Autodesk Inventor part; units mm, degrees
(part 3 of 3)
emboss "Emboss1" sketch "Sketch3" operation cut depth 0.1 direction (0, 1, 0) contours L352 L341 L342 L343 L344 L345 L346 L347 L348 L349 L350 L351 | S1 L0 L1 L2 S2 S3 S0 | L17 L6 L7 L8 L9 L10 L11 L12 L13 L14 L15 L16 | L22 L23 L24 L25 L26 L27 L28 L29 L30 L31 L32 L33 | L51 L52 L53 L54 L55 L56 L57 L58 L59 L60 L61 L62 | L63 L64 L65 L66 L67 L68 L69 L70 L71 L72 L73 L74 | L109 L98 L99 L100 L101 L102 L103 L104 L105 L106 L107 L108 | L128 L117 L118 L119 L120 L121 L122 L123 L124 L125 L126 L127 | L155 L144 L145 L146 L147 L148 L149 L150 L151 L152 L153 L154 | L167 L156 L157 L158 L159 L160 L161 L162 L163 L164 L165 L166 | L185 L186 L187 L188 L189 L190 L191 L192 L193 L194 L195 L196 | L218 L207 L208 L209 L210 L211 L212 L213 L214 L215 L216 L217 | L230 L219 L220 L221 L222 L223 L224 L225 L226 L227 L228 L229 | L242 L243 L244 L245 L246 L247 L248 L249 L250 L251 L252 L253 | L308 L297 L298 L299 L300 L301 L302 L303 L304 L305 L306 L307 | A0 L333 L334 L335 L336 L337 L338 L339 | A0 L313 L314 L315 L316 L317 L318 L319 | S155 S156 S157 S158 S159 L377 L378 S160 S161 S162 S163 S164 S153 S154 A0 | A0 S154 S155 | S152 S137 A0 | A0 S137 S138 S139 S140 S141 S142 L309 L310 S143 S144 S145 S146 S147 S148 S149 S150 L311 L312 S151 S152 | S132 S133 A0 | A0 S133 L290 L291 S134 S135 S136 L292 L293 L294 L295 L296 S132 | S8 L18 L19 S9 S10 S11 S12 S13 S14 S15 S16 L20 L21 S17 S18 S19 S20 S21 S22 S23 A0 | A0 S23 S8 | S120 S121 A0 | A0 S121 S122 S123 S124 S125 S118 S119 S120 | S24 S25 S26 S27 S28 S29 L34 L35 S30 S31 S32 S33 S34 S35 L36 L37 L38 L39 L40 S36 S37 A0 | A0 S37 S24 | S102 S89 A0 | A0 S89 S90 S91 S92 S93 S94 L264 L265 S95 S96 S97 S98 S99 S100 L266 L267 L268 L269 L270 S101 S102 | L112 L113 L114 L115 L116 L110 A0 | S81 S68 A0 | A0 S68 S69 S70 S71 S72 S73 L178 L179 S74 S75 S76 S77 S78 S79 L180 L181 L182 L183 L184 S80 S81 | S52 L140 L141 S53 S54 S55 S56 S57 S58 S59 S60 L142 L143 S61 S62 S63 S64 S65 S66 S67 A0 | A0 S67 S52 | L41 L42 L43 L44 L45 L46 L47 L48 L49 L50 | L75 L76 L77 L78 | L79 L80 L81 L82 | L83 L84 L85 L86 | L87 L88 L89 L90 L91 L92 L93 S38 S39 S40 L94 | L129 L130 L131 L132 L133 L134 L135 S45 S46 S47 L136 | L168 L169 L170 L171 L172 L173 L174 L175 L176 L177 | L197 L198 L199 L200 L201 L202 L203 L204 L205 L206 | L231 L232 L233 L234 L235 L236 L237 S82 S83 S84 L238 | L254 L255 L256 L257 L258 L259 L260 L261 L262 L263 | S103 S104 L271 L272 L273 L274 L275 S105 S106 | L279 L280 L281 L282 L283 L284 L285 S111 S112 S113 L286 | L321 L322 L323 L324 | L325 L326 L327 L328 | L329 L330 L331 L332 | L353 L354 L355 L356 L357 L358 L359 L360 | L364 L365 L366 L367 L368 L369 L370 L371 L372 L373 L374 L375 L376 | S172 L379 L380 S173 S174 S175 S176 S177 S178 S179 S180 L381 L382 S181 S182 S183 S184 S185 S186 S187 | L383 L384 L385 L386 L387 L388 L389 L390 | L398 L402 L403 L404 L405 L406 L407 L408 L409 L391 | L391 L402 L398 | L391 L392 L393 L394 L395 L396 L397 S188 S189 S190 L398 L402 | L413 L414 L415 L416 L417 L418 L419 L420 L421 L422 L423 L424 | L425 L426 L427 L428 L429 L430 L431 L432 L433 L434 | L435 L436 L437 L438 L439 L440 L441 L442 L443 L444 L445 L446 L447 | L448 L449 L450 L451 L452 L453 L454 L455 | L459 L460 L461 L462 L463 L464 L465 | L466 L467 L468 L469 L470 L471 L472 L473 L474 L475 L476 L477 | L478 L479 L480 L481 L482 L483 L484 S195 S196 S197 L485 | L489 L490 L491 L492 L493 L494 L495 L496 L497 L498 L499 L500 | S202 S203 L501 L502 L503 S204 S205 | S210 S211 L507 L508 L509 S212 S213 S214 S215 L510 L511 L512 S216 S217 | S218 S219 S220 S221 S222 S223 L513 L514 S224 S225 S226 S227 S228 S229 S230 S231 L515 L516 S232 S233 | L517 L518 L519 L520 L521 L522 L523 L524 L525 L526 L527 L528 | L529 L530 L531 L532 L533 L534 L535 S234 S235 S236 L536 | L540 L541 L542 L543 L544 L545 L546 L547 L548 L549 L550 L551 L552 | L553 L554 L555 L556 | L557 L558 L559 L560 | S241 L561 L562 L563 L564 L565 L566 L567 L568 L569 L570 L571 S242 S243 S244 L572 L573 S245 | L574 L575 S246 S247 S248 L576 L577 L578 L579 L580 S249 S250 L581 | S251 S252 S253 S254 S255 S256 L582 L583 S257 S258 S259 S260 S261 S262 S263 S264 L584 L585 S265 S266 | L586 L587 L588 L589 L590 L591 L592 S267 S268 S269 L593 | S274 S275 S276 S277 S278 S279 S280 S281 | S288 L597 L598 S289 S290 S291 S292 S293 S294 S295 S296 L599 L600 S297 S298 S299 S300 S301 S302 S303 | S304 L601 L602 S305 S306 S307 S308 S309 S310 S311 S312 L603 L604 S313 S314 S315 S316 S317 S318 S319 | L605 L606 L607 L608 L609 L610 L611 S320 S321 S322 L612 | S327 S328 S329 S330 S331 S332 S333 S334 | L616 L617 L618 L619 L620 L621 | L622 L623 L624 L625 L626 L627 | L628 L629 L630 L631 L632 L633 L634 L635 L636 L637 L638 L639 | L640 L641 L642 L643 L644 L645 L646 S341 S342 S343 L647 | S348 S349 L651 L652 L653 S350 S351 S352 L654 S353 | L661 L662 L663 L664 L665 L666 L667 L668 L669 L670 L671 L672 | L673 L674 L675 L676 L677 L678 L679 L680 | L684 L685 L686 L687 L688 L689 L690 S362 S363 S364 L691 | L695 L696 L697 L698 L699 L700 L701 L702 L703 L704 L705 L706 | L707 L708 L709 L710 L711 L712 L713 L714 L715 L716 | S369 S370 S371 S372 S373 S374 L717 L718 S375 S376 S377 S378 S379 S380 L719 L720 L721 L722 L723 S381 S382 | L724 L725 L726 L727 | L728 L729 L730 L731 | L732 L733 L734 L735 | S383 S384 S385 L736 S386 S387 S388 S389 L737 S390 S391 | S402 S403 S404 S405 S406 S407 S408 L738 L739 S409 S410 S411 S412 S413 | L740 L741 L742 L743 | L744 L745 L746 L747 | L748 L749 L750 L751 L752 L753 S421 L754 L755 L756 L757
equation "\"d2\" = Thickness"
equation "\"BendRadius\" = Thickness"
equation "\"BendReliefWidth\" = Thickness"
equation "\"BendReliefDepth\" = 0.5 * Thickness"
equation "\"CornerReliefSize\" = 4 * Thickness"
equation "\"MinimumRemnant\" = 2 * Thickness"
equation "\"TransitionRadius\" = BendRadius"
equation "\"JacobiRadiusSize\" = BendRadius"
equation "\"GapSize\" = Thickness"
equation "\"Thickness\" = 2"
body "Solid1"
